Autodesk Inventor part; units mm, degrees
(part 2 of 3)
  arc A208 (-48.5424, -4.4941) -> (-48.5247, -4.6815) centre (0, 0) ccw
  arc A209 (-48.7692, -5.0892) -> (-48.5247, -4.6815) centre (-48.9228, -4.7199) ccw
  spline S104 degree 3 poles (-48.7692, -5.0892) (-49.5171, -5.4153) (-50.0527, -5.68) (-50.6439, -6.0168) knots 0 0 0 0 1 1 1 1
  line L312 (-48.7692, -5.0892) -> (-49.5171, -5.4153) construction
  line L313 (-49.5171, -5.4153) -> (-50.0527, -5.68) construction
  line L314 (-50.0527, -5.68) -> (-50.6439, -6.0168) construction
  arc A210 (-50.6439, -6.0168) -> (-50.5492, -6.7669) centre (0, 0) ccw
  spline S105 degree 3 poles (-50.5492, -6.7669) (-49.8928, -6.946) (-49.3082, -7.0693) (-48.5027, -7.1991) knots 0 0 0 0 1 1 1 1
  line L315 (-50.5492, -6.7669) -> (-49.8928, -6.946) construction
  line L316 (-49.8928, -6.946) -> (-49.3082, -7.0693) construction
  line L317 (-49.3082, -7.0693) -> (-48.5027, -7.1991) construction
  arc A211 (-48.1644, -7.5332) -> (-48.5027, -7.1991) centre (-48.5596, -7.595) ccw
  arc A212 (-48.1644, -7.5332) -> (-48.135, -7.7191) centre (0, 0) ccw
  arc A213 (-48.3535, -8.1414) -> (-48.135, -7.7191) centre (-48.5299, -7.7825) ccw
  spline S106 degree 3 poles (-48.3535, -8.1414) (-49.0794, -8.5138) (-49.5973, -8.8117) (-50.1662, -9.1848) knots 0 0 0 0 1 1 1 1
  line L318 (-48.3535, -8.1414) -> (-49.0794, -8.5138) construction
  line L319 (-49.0794, -8.5138) -> (-49.5973, -8.8117) construction
  line L320 (-49.5973, -8.8117) -> (-50.1662, -9.1848) construction
  arc A214 (-50.1662, -9.1848) -> (-50.0245, -9.9276) centre (0, 0) ccw
  spline S107 degree 3 poles (-50.0245, -9.9276) (-49.3582, -10.0651) (-48.767, -10.1514) (-47.955, -10.2304) knots 0 0 0 0 1 1 1 1
  line L321 (-50.0245, -9.9276) -> (-49.3582, -10.0651) construction
  line L322 (-49.3582, -10.0651) -> (-48.767, -10.1514) construction
  line L323 (-48.767, -10.1514) -> (-47.955, -10.2304) construction
  arc A215 (-47.5964, -10.5426) -> (-47.955, -10.2304) centre (-47.9869, -10.6291) ccw
  arc A216 (-47.5964, -10.5426) -> (-47.5553, -10.7263) centre (0, 0) ccw
  arc A217 (-47.7468, -11.1615) -> (-47.5553, -10.7263) centre (-47.9455, -10.8143) ccw
  spline S108 degree 3 poles (-47.7468, -11.1615) (-48.448, -11.5787) (-48.9462, -11.9085) (-49.4905, -12.3167) knots 0 0 0 0 1 1 1 1
  line L324 (-47.7468, -11.1615) -> (-48.448, -11.5787) construction
  line L325 (-48.448, -11.5787) -> (-48.9462, -11.9085) construction
  line L326 (-48.9462, -11.9085) -> (-49.4905, -12.3167) construction
  arc A218 (-49.4905, -12.3167) -> (-49.3024, -13.049) centre (0, 0) ccw
  spline S109 degree 3 poles (-49.3024, -13.049) (-48.6288, -13.1445) (-48.0334, -13.1935) (-47.218, -13.2213) knots 0 0 0 0 1 1 1 1
  line L327 (-49.3024, -13.049) -> (-48.6288, -13.1445) construction
  line L328 (-48.6288, -13.1445) -> (-48.0334, -13.1935) construction
  line L329 (-48.0334, -13.1935) -> (-47.218, -13.2213) construction
  arc A219 (-46.8405, -13.5104) -> (-47.218, -13.2213) centre (-47.2248, -13.6213) ccw
  arc A220 (-46.8405, -13.5104) -> (-46.788, -13.6912) centre (0, 0) ccw
  arc A221 (-46.9518, -14.1375) -> (-46.788, -13.6912) centre (-47.1719, -13.8035) ccw
  spline S110 degree 3 poles (-46.9518, -14.1375) (-47.6253, -14.5979) (-48.1018, -14.9584) (-48.6194, -15.3999) knots 0 0 0 0 1 1 1 1
  line L330 (-46.9518, -14.1375) -> (-47.6253, -14.5979) construction
  line L331 (-47.6253, -14.5979) -> (-48.1018, -14.9584) construction
  line L332 (-48.1018, -14.9584) -> (-48.6194, -15.3999) construction
  arc A222 (-48.6194, -15.3999) -> (-48.3858, -16.119) centre (0, 0) ccw
  spline S111 degree 3 poles (-48.3858, -16.119) (-47.7075, -16.172) (-47.1102, -16.1835) (-46.2946, -16.1601) knots 0 0 0 0 1 1 1 1
  line L333 (-48.3858, -16.119) -> (-47.7075, -16.172) construction
  line L334 (-47.7075, -16.172) -> (-47.1102, -16.1835) construction
  line L335 (-47.1102, -16.1835) -> (-46.2946, -16.1601) construction
  arc A223 (-45.8997, -16.4249) -> (-46.2946, -16.1601) centre (-46.2763, -16.5596) ccw
  arc A224 (-45.8997, -16.4249) -> (-45.836, -16.602) centre (0, 0) ccw
  arc A225 (-45.9714, -17.0578) -> (-45.836, -16.602) centre (-46.2121, -16.7382) ccw
  spline S112 degree 3 poles (-45.9714, -17.0578) (-46.6147, -17.5595) (-47.0677, -17.9492) (-47.5565, -18.4224) knots 0 0 0 0 1 1 1 1
  line L336 (-45.9714, -17.0578) -> (-46.6147, -17.5595) construction
  line L337 (-46.6147, -17.5595) -> (-47.0677, -17.9492) construction
  line L338 (-47.0677, -17.9492) -> (-47.5565, -18.4224) construction
  arc A226 (-47.5565, -18.4224) -> (-47.2782, -19.1254) centre (0, 0) ccw
  spline S113 degree 3 poles (-47.2782, -19.1254) (-46.5979, -19.1356) (-46.001, -19.1096) (-45.1886, -19.035) knots 0 0 0 0 1 1 1 1
  line L339 (-47.2782, -19.1254) -> (-46.5979, -19.1356) construction
  line L340 (-46.5979, -19.1356) -> (-46.001, -19.1096) construction
  line L341 (-46.001, -19.1096) -> (-45.1886, -19.035) construction
  arc A227 (-44.7778, -19.2745) -> (-45.1886, -19.035) centre (-45.1452, -19.4327) ccw
  arc A228 (-44.7778, -19.2745) -> (-44.7031, -19.4473) centre (0, 0) ccw
  arc A229 (-44.8097, -19.9107) -> (-44.7031, -19.4473) centre (-45.0699, -19.6069) ccw
  spline S114 degree 3 poles (-44.8097, -19.9107) (-45.4202, -20.4519) (-45.8478, -20.8692) (-46.3059, -21.3721) knots 0 0 0 0 1 1 1 1
  line L342 (-44.8097, -19.9107) -> (-45.4202, -20.4519) construction
  line L343 (-45.4202, -20.4519) -> (-45.8478, -20.8692) construction
  line L344 (-45.8478, -20.8692) -> (-46.3059, -21.3721) construction
  arc A230 (-46.3059, -21.3721) -> (-45.984, -22.0563) centre (0, 0) ccw
  spline S115 degree 3 poles (-45.984, -22.0563) (-45.3044, -22.0238) (-44.7103, -21.9604) (-43.9042, -21.8349) knots 0 0 0 0 1 1 1 1
  line L345 (-45.984, -22.0563) -> (-45.3044, -22.0238) construction
  line L346 (-45.3044, -22.0238) -> (-44.7103, -21.9604) construction
  line L347 (-44.7103, -21.9604) -> (-43.9042, -21.8349) construction
  arc A231 (-43.4792, -22.0481) -> (-43.9042, -21.8349) centre (-43.836, -22.229) ccw
  arc A232 (-43.4792, -22.0481) -> (-43.3938, -22.2159) centre (0, 0) ccw
  arc A233 (-43.471, -22.685) -> (-43.3938, -22.2159) centre (-43.7498, -22.3981) ccw
  spline S116 degree 3 poles (-43.471, -22.685) (-44.0464, -23.2635) (-44.4469, -23.7068) (-44.8726, -24.2375) knots 0 0 0 0 1 1 1 1
  line L348 (-43.471, -22.685) -> (-44.0464, -23.2635) construction
  line L349 (-44.0464, -23.2635) -> (-44.4469, -23.7068) construction
  line L350 (-44.4469, -23.7068) -> (-44.8726, -24.2375) construction
  arc A234 (-44.8726, -24.2375) -> (-44.5083, -24.9001) centre (0, 0) ccw
  spline S117 degree 3 poles (-44.5083, -24.9001) (-43.8322, -24.825) (-43.2432, -24.7244) (-42.4465, -24.5486) knots 0 0 0 0 1 1 1 1
  line L351 (-44.5083, -24.9001) -> (-43.8322, -24.825) construction
  line L352 (-43.8322, -24.825) -> (-43.2432, -24.7244) construction
  line L353 (-43.2432, -24.7244) -> (-42.4465, -24.5486) construction
  arc A235 (-42.009, -24.7347) -> (-42.4465, -24.5486) centre (-42.3537, -24.9377) ccw
  arc A236 (-42.009, -24.7347) -> (-41.9132, -24.8967) centre (0, 0) ccw
  arc A237 (-41.9609, -25.3698) -> (-41.9132, -24.8967) centre (-42.2571, -25.101) ccw
  spline S118 degree 3 poles (-41.9609, -25.3698) (-42.4987, -25.9832) (-42.8706, -26.4509) (-43.2622, -27.0072) knots 0 0 0 0 1 1 1 1
  line L354 (-41.9609, -25.3698) -> (-42.4987, -25.9832) construction
  line L355 (-42.4987, -25.9832) -> (-42.8706, -26.4509) construction
  line L356 (-42.8706, -26.4509) -> (-43.2622, -27.0072) construction
  arc A238 (-43.2622, -27.0072) -> (-42.857, -27.6457) centre (0, 0) ccw
  spline S119 degree 3 poles (-42.857, -27.6457) (-42.1869, -27.5283) (-41.6054, -27.3909) (-40.8213, -27.1654) knots 0 0 0 0 1 1 1 1
  line L357 (-42.857, -27.6457) -> (-42.1869, -27.5283) construction
  line L358 (-42.1869, -27.5283) -> (-41.6054, -27.3909) construction
  line L359 (-41.6054, -27.3909) -> (-40.8213, -27.1654) construction
  arc A239 (-40.373, -27.3237) -> (-40.8213, -27.1654) centre (-40.7043, -27.5479) ccw
  arc A240 (-40.373, -27.3237) -> (-40.2672, -27.4794) centre (0, 0) ccw
  arc A241 (-40.2851, -27.9545) -> (-40.2672, -27.4794) centre (-40.5976, -27.7048) ccw
  spline S120 degree 3 poles (-40.2851, -27.9545) (-40.7834, -28.6005) (-41.1252, -29.0905) (-41.481, -29.6704) knots 0 0 0 0 1 1 1 1
  line L360 (-40.2851, -27.9545) -> (-40.7834, -28.6005) construction
  line L361 (-40.7834, -28.6005) -> (-41.1252, -29.0905) construction
  line L362 (-41.1252, -29.0905) -> (-41.481, -29.6704) construction
  arc A242 (-41.481, -29.6704) -> (-41.0366, -30.2821) centre (0, 0) ccw
  spline S121 degree 3 poles (-41.0366, -30.2821) (-40.3751, -30.1229) (-39.8034, -29.9493) (-39.0351, -29.675) knots 0 0 0 0 1 1 1 1
  line L363 (-41.0366, -30.2821) -> (-40.3751, -30.1229) construction
  line L364 (-40.3751, -30.1229) -> (-39.8034, -29.9493) construction
  line L365 (-39.8034, -29.9493) -> (-39.0351, -29.675) construction
  arc A243 (-38.5777, -29.8048) -> (-39.0351, -29.675) centre (-38.8942, -30.0493) ccw
  arc A244 (-38.5777, -29.8048) -> (-38.4623, -29.9535) centre (0, 0) ccw
  arc A245 (-38.4503, -30.4288) -> (-38.4623, -29.9535) centre (-38.7779, -30.1993) ccw
  spline S122 degree 3 poles (-38.4503, -30.4288) (-38.9071, -31.1049) (-39.2174, -31.6154) (-39.5361, -32.2165) knots 0 0 0 0 1 1 1 1
  line L366 (-38.4503, -30.4288) -> (-38.9071, -31.1049) construction
  line L367 (-38.9071, -31.1049) -> (-39.2174, -31.6154) construction
  line L368 (-39.2174, -31.6154) -> (-39.5361, -32.2165) construction
  arc A246 (-39.5361, -32.2165) -> (-39.0542, -32.7991) centre (0, 0) ccw
  spline S123 degree 3 poles (-39.0542, -32.7991) (-38.404, -32.5986) (-37.8444, -32.3894) (-37.0947, -32.0674) knots 0 0 0 0 1 1 1 1
  line L369 (-39.0542, -32.7991) -> (-38.404, -32.5986) construction
  line L370 (-38.404, -32.5986) -> (-37.8444, -32.3894) construction
  line L371 (-37.8444, -32.3894) -> (-37.0947, -32.0674) construction
  arc A247 (-36.6301, -32.1683) -> (-37.0947, -32.0674) centre (-36.9306, -32.4322) ccw
  arc A248 (-36.6301, -32.1683) -> (-36.5056, -32.3095) centre (0, 0) ccw
  arc A249 (-36.4638, -32.7831) -> (-36.5056, -32.3095) centre (-36.8051, -32.5746) ccw
  spline S124 degree 3 poles (-36.4638, -32.7831) (-36.8772, -33.4865) (-37.1549, -34.0155) (-37.4352, -34.6354) knots 0 0 0 0 1 1 1 1
  line L372 (-36.4638, -32.7831) -> (-36.8772, -33.4865) construction
  line L373 (-36.8772, -33.4865) -> (-37.1549, -34.0155) construction
  line L374 (-37.1549, -34.0155) -> (-37.4352, -34.6354) construction
  arc A250 (-37.4352, -34.6354) -> (-36.9176, -35.1866) centre (0, 0) ccw
  spline S125 degree 3 poles (-36.9176, -35.1866) (-36.2814, -34.9457) (-35.7359, -34.7018) (-35.008, -34.3334) knots 0 0 0 0 1 1 1 1
  line L375 (-36.9176, -35.1866) -> (-36.2814, -34.9457) construction
  line L376 (-36.2814, -34.9457) -> (-35.7359, -34.7018) construction
  line L377 (-35.7359, -34.7018) -> (-35.008, -34.3334) construction
  arc A251 (-34.538, -34.4048) -> (-35.008, -34.3334) centre (-34.8213, -34.6871) ccw
  arc A252 (-34.538, -34.4048) -> (-34.4048, -34.538) centre (0, 0) ccw
  arc A253 (-34.3334, -35.008) -> (-34.4048, -34.538) centre (-34.6871, -34.8213) ccw
  spline S126 degree 3 poles (-34.3334, -35.008) (-34.7018, -35.7359) (-34.9457, -36.2814) (-35.1866, -36.9176) knots 0 0 0 0 1 1 1 1
  line L378 (-34.3334, -35.008) -> (-34.7018, -35.7359) construction
  line L379 (-34.7018, -35.7359) -> (-34.9457, -36.2814) construction
  line L380 (-34.9457, -36.2814) -> (-35.1866, -36.9176) construction
  arc A254 (-35.1866, -36.9176) -> (-34.6354, -37.4352) centre (0, 0) ccw
  spline S127 degree 3 poles (-34.6354, -37.4352) (-34.0155, -37.1549) (-33.4865, -36.8772) (-32.7831, -36.4638) knots 0 0 0 0 1 1 1 1
  line L381 (-34.6354, -37.4352) -> (-34.0155, -37.1549) construction
  line L382 (-34.0155, -37.1549) -> (-33.4865, -36.8772) construction
  line L383 (-33.4865, -36.8772) -> (-32.7831, -36.4638) construction
  arc A255 (-32.3095, -36.5056) -> (-32.7831, -36.4638) centre (-32.5746, -36.8051) ccw
  arc A256 (-32.3095, -36.5056) -> (-32.1683, -36.6301) centre (0, 0) ccw
  arc A257 (-32.0674, -37.0947) -> (-32.1683, -36.6301) centre (-32.4322, -36.9306) ccw
  spline S128 degree 3 poles (-32.0674, -37.0947) (-32.3894, -37.8444) (-32.5986, -38.404) (-32.7991, -39.0542) knots 0 0 0 0 1 1 1 1
  line L384 (-32.0674, -37.0947) -> (-32.3894, -37.8444) construction
  line L385 (-32.3894, -37.8444) -> (-32.5986, -38.404) construction
  line L386 (-32.5986, -38.404) -> (-32.7991, -39.0542) construction
  arc A258 (-32.7991, -39.0542) -> (-32.2165, -39.5361) centre (0, 0) ccw
  spline S129 degree 3 poles (-32.2165, -39.5361) (-31.6154, -39.2174) (-31.1049, -38.9071) (-30.4288, -38.4503) knots 0 0 0 0 1 1 1 1
  line L387 (-32.2165, -39.5361) -> (-31.6154, -39.2174) construction
  line L388 (-31.6154, -39.2174) -> (-31.1049, -38.9071) construction
  line L389 (-31.1049, -38.9071) -> (-30.4288, -38.4503) construction
  arc A259 (-29.9535, -38.4623) -> (-30.4288, -38.4503) centre (-30.1993, -38.7779) ccw
  arc A260 (-29.9535, -38.4623) -> (-29.8048, -38.5777) centre (0, 0) ccw
  arc A261 (-29.675, -39.0351) -> (-29.8048, -38.5777) centre (-30.0493, -38.8942) ccw
  spline S130 degree 3 poles (-29.675, -39.0351) (-29.9493, -39.8034) (-30.1229, -40.3751) (-30.2821, -41.0366) knots 0 0 0 0 1 1 1 1
  line L390 (-29.675, -39.0351) -> (-29.9493, -39.8034) construction
  line L391 (-29.9493, -39.8034) -> (-30.1229, -40.3751) construction
  line L392 (-30.1229, -40.3751) -> (-30.2821, -41.0366) construction
  arc A262 (-30.2821, -41.0366) -> (-29.6704, -41.481) centre (0, 0) ccw
  spline S131 degree 3 poles (-29.6704, -41.481) (-29.0905, -41.1252) (-28.6005, -40.7834) (-27.9545, -40.2851) knots 0 0 0 0 1 1 1 1
  line L393 (-29.6704, -41.481) -> (-29.0905, -41.1252) construction
  line L394 (-29.0905, -41.1252) -> (-28.6005, -40.7834) construction
  line L395 (-28.6005, -40.7834) -> (-27.9545, -40.2851) construction
  arc A263 (-27.4794, -40.2672) -> (-27.9545, -40.2851) centre (-27.7048, -40.5976) ccw
  arc A264 (-27.4794, -40.2672) -> (-27.3237, -40.373) centre (0, 0) ccw
  arc A265 (-27.1654, -40.8213) -> (-27.3237, -40.373) centre (-27.5479, -40.7043) ccw
  spline S132 degree 3 poles (-27.1654, -40.8213) (-27.3909, -41.6054) (-27.5283, -42.1869) (-27.6457, -42.857) knots 0 0 0 0 1 1 1 1
  line L396 (-27.1654, -40.8213) -> (-27.3909, -41.6054) construction
  line L397 (-27.3909, -41.6054) -> (-27.5283, -42.1869) construction
  line L398 (-27.5283, -42.1869) -> (-27.6457, -42.857) construction
  arc A266 (-27.6457, -42.857) -> (-27.0072, -43.2622) centre (0, 0) ccw
  spline S133 degree 3 poles (-27.0072, -43.2622) (-26.4509, -42.8706) (-25.9832, -42.4987) (-25.3698, -41.9609) knots 0 0 0 0 1 1 1 1
  line L399 (-27.0072, -43.2622) -> (-26.4509, -42.8706) construction
  line L400 (-26.4509, -42.8706) -> (-25.9832, -42.4987) construction
  line L401 (-25.9832, -42.4987) -> (-25.3698, -41.9609) construction
  arc A267 (-24.8967, -41.9132) -> (-25.3698, -41.9609) centre (-25.101, -42.2571) ccw
  arc A268 (-24.8967, -41.9132) -> (-24.7347, -42.009) centre (0, 0) ccw
  arc A269 (-24.5486, -42.4465) -> (-24.7347, -42.009) centre (-24.9377, -42.3537) ccw
  spline S134 degree 3 poles (-24.5486, -42.4465) (-24.7244, -43.2432) (-24.825, -43.8322) (-24.9001, -44.5083) knots 0 0 0 0 1 1 1 1
  line L402 (-24.5486, -42.4465) -> (-24.7244, -43.2432) construction
  line L403 (-24.7244, -43.2432) -> (-24.825, -43.8322) construction
  line L404 (-24.825, -43.8322) -> (-24.9001, -44.5083) construction
  arc A270 (-24.9001, -44.5083) -> (-24.2375, -44.8726) centre (0, 0) ccw
  spline S135 degree 3 poles (-24.2375, -44.8726) (-23.7068, -44.4469) (-23.2635, -44.0464) (-22.685, -43.471) knots 0 0 0 0 1 1 1 1
  line L405 (-24.2375, -44.8726) -> (-23.7068, -44.4469) construction
  line L406 (-23.7068, -44.4469) -> (-23.2635, -44.0464) construction
  line L407 (-23.2635, -44.0464) -> (-22.685, -43.471) construction
  arc A271 (-22.2159, -43.3938) -> (-22.685, -43.471) centre (-22.3981, -43.7498) ccw
  arc A272 (-22.2159, -43.3938) -> (-22.0481, -43.4792) centre (0, 0) ccw
  arc A273 (-21.8349, -43.9042) -> (-22.0481, -43.4792) centre (-22.229, -43.836) ccw
  spline S136 degree 3 poles (-21.8349, -43.9042) (-21.9604, -44.7103) (-22.0238, -45.3044) (-22.0563, -45.984) knots 0 0 0 0 1 1 1 1
  line L408 (-21.8349, -43.9042) -> (-21.9604, -44.7103) construction
  line L409 (-21.9604, -44.7103) -> (-22.0238, -45.3044) construction
  line L410 (-22.0238, -45.3044) -> (-22.0563, -45.984) construction
  arc A274 (-22.0563, -45.984) -> (-21.3721, -46.3059) centre (0, 0) ccw
  spline S137 degree 3 poles (-21.3721, -46.3059) (-20.8692, -45.8478) (-20.4519, -45.4202) (-19.9107, -44.8097) knots 0 0 0 0 1 1 1 1
  line L411 (-21.3721, -46.3059) -> (-20.8692, -45.8478) construction
  line L412 (-20.8692, -45.8478) -> (-20.4519, -45.4202) construction
  line L413 (-20.4519, -45.4202) -> (-19.9107, -44.8097) construction
  arc A275 (-19.4473, -44.7031) -> (-19.9107, -44.8097) centre (-19.6069, -45.0699) ccw
  arc A276 (-19.4473, -44.7031) -> (-19.2745, -44.7778) centre (0, 0) ccw
  arc A277 (-19.035, -45.1886) -> (-19.2745, -44.7778) centre (-19.4327, -45.1452) ccw
  spline S138 degree 3 poles (-19.035, -45.1886) (-19.1096, -46.001) (-19.1356, -46.5979) (-19.1254, -47.2782) knots 0 0 0 0 1 1 1 1
  line L414 (-19.035, -45.1886) -> (-19.1096, -46.001) construction
  line L415 (-19.1096, -46.001) -> (-19.1356, -46.5979) construction
  line L416 (-19.1356, -46.5979) -> (-19.1254, -47.2782) construction
  arc A278 (-19.1254, -47.2782) -> (-18.4224, -47.5565) centre (0, 0) ccw
  spline S139 degree 3 poles (-18.4224, -47.5565) (-17.9492, -47.0677) (-17.5595, -46.6147) (-17.0578, -45.9714) knots 0 0 0 0 1 1 1 1
  line L417 (-18.4224, -47.5565) -> (-17.9492, -47.0677) construction
  line L418 (-17.9492, -47.0677) -> (-17.5595, -46.6147) construction
  line L419 (-17.5595, -46.6147) -> (-17.0578, -45.9714) construction
  arc A279 (-16.602, -45.836) -> (-17.0578, -45.9714) centre (-16.7382, -46.2121) ccw
  arc A280 (-16.602, -45.836) -> (-16.4249, -45.8997) centre (0, 0) ccw
  arc A281 (-16.1601, -46.2946) -> (-16.4249, -45.8997) centre (-16.5596, -46.2763) ccw
  spline S140 degree 3 poles (-16.1601, -46.2946) (-16.1835, -47.1102) (-16.172, -47.7075) (-16.119, -48.3858) knots 0 0 0 0 1 1 1 1
  line L420 (-16.1601, -46.2946) -> (-16.1835, -47.1102) construction
  line L421 (-16.1835, -47.1102) -> (-16.172, -47.7075) construction
  line L422 (-16.172, -47.7075) -> (-16.119, -48.3858) construction
  arc A282 (-16.119, -48.3858) -> (-15.3999, -48.6194) centre (0, 0) ccw
  spline S141 degree 3 poles (-15.3999, -48.6194) (-14.9584, -48.1018) (-14.5979, -47.6253) (-14.1375, -46.9518) knots 0 0 0 0 1 1 1 1
  line L423 (-15.3999, -48.6194) -> (-14.9584, -48.1018) construction
  line L424 (-14.9584, -48.1018) -> (-14.5979, -47.6253) construction
  line L425 (-14.5979, -47.6253) -> (-14.1375, -46.9518) construction
  arc A283 (-13.6912, -46.788) -> (-14.1375, -46.9518) centre (-13.8035, -47.1719) ccw
  arc A284 (-13.6912, -46.788) -> (-13.5104, -46.8405) centre (0, 0) ccw
  arc A285 (-13.2213, -47.218) -> (-13.5104, -46.8405) centre (-13.6213, -47.2248) ccw
  spline S142 degree 3 poles (-13.2213, -47.218) (-13.1935, -48.0334) (-13.1445, -48.6288) (-13.049, -49.3024) knots 0 0 0 0 1 1 1 1
  line L426 (-13.2213, -47.218) -> (-13.1935, -48.0334) construction
  line L427 (-13.1935, -48.0334) -> (-13.1445, -48.6288) construction
  line L428 (-13.1445, -48.6288) -> (-13.049, -49.3024) construction
  arc A286 (-13.049, -49.3024) -> (-12.3167, -49.4905) centre (0, 0) ccw
  spline S143 degree 3 poles (-12.3167, -49.4905) (-11.9085, -48.9462) (-11.5787, -48.448) (-11.1615, -47.7468) knots 0 0 0 0 1 1 1 1
  line L429 (-12.3167, -49.4905) -> (-11.9085, -48.9462) construction
  line L430 (-11.9085, -48.9462) -> (-11.5787, -48.448) construction
  line L431 (-11.5787, -48.448) -> (-11.1615, -47.7468) construction
  arc A287 (-10.7263, -47.5553) -> (-11.1615, -47.7468) centre (-10.8143, -47.9455) ccw
  arc A288 (-10.7263, -47.5553) -> (-10.5426, -47.5964) centre (0, 0) ccw
  arc A289 (-10.2304, -47.955) -> (-10.5426, -47.5964) centre (-10.6291, -47.9869) ccw
  spline S144 degree 3 poles (-10.2304, -47.955) (-10.1514, -48.767) (-10.0651, -49.3582) (-9.9276, -50.0245) knots 0 0 0 0 1 1 1 1
  line L432 (-10.2304, -47.955) -> (-10.1514, -48.767) construction
  line L433 (-10.1514, -48.767) -> (-10.0651, -49.3582) construction
  line L434 (-10.0651, -49.3582) -> (-9.9276, -50.0245) construction
  arc A290 (-9.9276, -50.0245) -> (-9.1848, -50.1662) centre (0, 0) ccw
  spline S145 degree 3 poles (-9.1848, -50.1662) (-8.8117, -49.5973) (-8.5138, -49.0794) (-8.1414, -48.3535) knots 0 0 0 0 1 1 1 1
  line L435 (-9.1848, -50.1662) -> (-8.8117, -49.5973) construction
  line L436 (-8.8117, -49.5973) -> (-8.5138, -49.0794) construction
  line L437 (-8.5138, -49.0794) -> (-8.1414, -48.3535) construction
  arc A291 (-7.7191, -48.135) -> (-8.1414, -48.3535) centre (-7.7825, -48.5299) ccw
  arc A292 (-7.7191, -48.135) -> (-7.5332, -48.1644) centre (0, 0) ccw
  arc A293 (-7.1991, -48.5027) -> (-7.5332, -48.1644) centre (-7.595, -48.5596) ccw
  spline S146 degree 3 poles (-7.1991, -48.5027) (-7.0693, -49.3082) (-6.946, -49.8928) (-6.7669, -50.5492) knots 0 0 0 0 1 1 1 1
  line L438 (-7.1991, -48.5027) -> (-7.0693, -49.3082) construction
  line L439 (-7.0693, -49.3082) -> (-6.946, -49.8928) construction
  line L440 (-6.946, -49.8928) -> (-6.7669, -50.5492) construction
  arc A294 (-6.7669, -50.5492) -> (-6.0168, -50.6439) centre (0, 0) ccw
  spline S147 degree 3 poles (-6.0168, -50.6439) (-5.68, -50.0527) (-5.4153, -49.5171) (-5.0892, -48.7692) knots 0 0 0 0 1 1 1 1
  line L441 (-6.0168, -50.6439) -> (-5.68, -50.0527) construction
  line L442 (-5.68, -50.0527) -> (-5.4153, -49.5171) construction
  line L443 (-5.4153, -49.5171) -> (-5.0892, -48.7692) construction
  arc A295 (-4.6815, -48.5247) -> (-5.0892, -48.7692) centre (-4.7199, -48.9228) ccw
  arc A296 (-4.6815, -48.5247) -> (-4.4941, -48.5424) centre (0, 0) ccw
  arc A297 (-4.1394, -48.859) -> (-4.4941, -48.5424) centre (-4.5309, -48.9407) ccw
  spline S148 degree 3 poles (-4.1394, -48.859) (-3.9592, -49.6548) (-3.7995, -50.2305) (-3.5795, -50.8743) knots 0 0 0 0 1 1 1 1
  line L444 (-4.1394, -48.859) -> (-3.9592, -49.6548) construction
  line L445 (-3.9592, -49.6548) -> (-3.7995, -50.2305) construction
  line L446 (-3.7995, -50.2305) -> (-3.5795, -50.8743) construction
  arc A298 (-3.5795, -50.8743) -> (-2.8249, -50.9218) centre (0, 0) ccw
  spline S149 degree 3 poles (-2.8249, -50.9218) (-2.526, -50.3106) (-2.2954, -49.7595) (-2.0169, -48.9926) knots 0 0 0 0 1 1 1 1
  line L447 (-2.8249, -50.9218) -> (-2.526, -50.3106) construction
  line L448 (-2.526, -50.3106) -> (-2.2954, -49.7595) construction
  line L449 (-2.2954, -49.7595) -> (-2.0169, -48.9926) construction
  arc A299 (-1.6254, -48.7229) -> (-2.0169, -48.9926) centre (-1.6387, -49.1227) ccw
  arc A300 (-1.6254, -48.7229) -> (-1.4372, -48.7288) centre (0, 0) ccw
  arc A301 (-1.0633, -49.0225) -> (-1.4372, -48.7288) centre (-1.449, -49.1286) ccw
  spline S150 degree 3 poles (-1.0633, -49.0225) (-0.8336, -49.8054) (-0.638, -50.3699) (-0.3781, -50.9987) knots 0 0 0 0 1 1 1 1
  line L450 (-1.0633, -49.0225) -> (-0.8336, -49.8054) construction
  line L451 (-0.8336, -49.8054) -> (-0.638, -50.3699) construction
  line L452 (-0.638, -50.3699) -> (-0.3781, -50.9987) construction
  arc A302 (-0.3781, -50.9987) -> (0.3781, -50.9987) centre (0, 0) ccw
  spline S151 degree 3 poles (0.3781, -50.9987) (0.638, -50.3699) (0.8336, -49.8054) (1.0633, -49.0225) knots 0 0 0 0 1 1 1 1
  line L453 (0.3781, -50.9987) -> (0.638, -50.3699) construction
  line L454 (0.638, -50.3699) -> (0.8336, -49.8054) construction
  line L455 (0.8336, -49.8054) -> (1.0633, -49.0225) construction
  arc A303 (1.4372, -48.7288) -> (1.0633, -49.0225) centre (1.449, -49.1286) ccw
  arc A304 (1.4372, -48.7288) -> (1.6254, -48.7229) centre (0, 0) ccw
  arc A305 (2.0169, -48.9926) -> (1.6254, -48.7229) centre (1.6387, -49.1227) ccw
  spline S152 degree 3 poles (2.0169, -48.9926) (2.2954, -49.7595) (2.526, -50.3106) (2.8249, -50.9218) knots 0 0 0 0 1 1 1 1
  line L456 (2.0169, -48.9926) -> (2.2954, -49.7595) construction
  line L457 (2.2954, -49.7595) -> (2.526, -50.3106) construction
  line L458 (2.526, -50.3106) -> (2.8249, -50.9218) construction
  arc A306 (2.8249, -50.9218) -> (3.5795, -50.8743) centre (0, 0) ccw
  spline S153 degree 3 poles (3.5795, -50.8743) (3.7995, -50.2305) (3.9592, -49.6548) (4.1394, -48.859) knots 0 0 0 0 1 1 1 1
  line L459 (3.5795, -50.8743) -> (3.7995, -50.2305) construction
  line L460 (3.7995, -50.2305) -> (3.9592, -49.6548) construction
  line L461 (3.9592, -49.6548) -> (4.1394, -48.859) construction
  arc A307 (4.4941, -48.5424) -> (4.1394, -48.859) centre (4.5309, -48.9407) ccw
  arc A308 (4.4941, -48.5424) -> (4.6815, -48.5247) centre (0, 0) ccw
  arc A309 (5.0892, -48.7692) -> (4.6815, -48.5247) centre (4.7199, -48.9228) ccw
  spline S154 degree 3 poles (5.0892, -48.7692) (5.4153, -49.5171) (5.68, -50.0527) (6.0168, -50.6439) knots 0 0 0 0 1 1 1 1
  line L462 (5.0892, -48.7692) -> (5.4153, -49.5171) construction
  line L463 (5.4153, -49.5171) -> (5.68, -50.0527) construction
  line L464 (5.68, -50.0527) -> (6.0168, -50.6439) construction
  arc A310 (6.0168, -50.6439) -> (6.7669, -50.5492) centre (0, 0) ccw
  spline S155 degree 3 poles (6.7669, -50.5492) (6.946, -49.8928) (7.0693, -49.3082) (7.1991, -48.5027) knots 0 0 0 0 1 1 1 1
  line L465 (6.7669, -50.5492) -> (6.946, -49.8928) construction
  line L466 (6.946, -49.8928) -> (7.0693, -49.3082) construction
  line L467 (7.0693, -49.3082) -> (7.1991, -48.5027) construction
  arc A311 (7.5332, -48.1644) -> (7.1991, -48.5027) centre (7.595, -48.5596) ccw
  arc A312 (7.5332, -48.1644) -> (7.7191, -48.135) centre (0, 0) ccw
  arc A313 (8.1414, -48.3535) -> (7.7191, -48.135) centre (7.7825, -48.5299) ccw
  spline S156 degree 3 poles (8.1414, -48.3535) (8.5138, -49.0794) (8.8117, -49.5973) (9.1848, -50.1662) knots 0 0 0 0 1 1 1 1
  line L468 (8.1414, -48.3535) -> (8.5138, -49.0794) construction
  line L469 (8.5138, -49.0794) -> (8.8117, -49.5973) construction
  line L470 (8.8117, -49.5973) -> (9.1848, -50.1662) construction
  arc A314 (9.1848, -50.1662) -> (9.9276, -50.0245) centre (0, 0) ccw
  spline S157 degree 3 poles (9.9276, -50.0245) (10.0651, -49.3582) (10.1514, -48.767) (10.2304, -47.955) knots 0 0 0 0 1 1 1 1
  line L471 (9.9276, -50.0245) -> (10.0651, -49.3582) construction
  line L472 (10.0651, -49.3582) -> (10.1514, -48.767) construction
  line L473 (10.1514, -48.767) -> (10.2304, -47.955) construction
  arc A315 (10.5426, -47.5964) -> (10.2304, -47.955) centre (10.6291, -47.9869) ccw
  arc A316 (10.5426, -47.5964) -> (10.7263, -47.5553) centre (0, 0) ccw
  arc A317 (11.1615, -47.7468) -> (10.7263, -47.5553) centre (10.8143, -47.9455) ccw
  spline S158 degree 3 poles (11.1615, -47.7468) (11.5787, -48.448) (11.9085, -48.9462) (12.3167, -49.4905) knots 0 0 0 0 1 1 1 1
  line L474 (11.1615, -47.7468) -> (11.5787, -48.448) construction
  line L475 (11.5787, -48.448) -> (11.9085, -48.9462) construction
  line L476 (11.9085, -48.9462) -> (12.3167, -49.4905) construction
  arc A318 (12.3167, -49.4905) -> (13.049, -49.3024) centre (0, 0) ccw
  spline S159 degree 3 poles (13.049, -49.3024) (13.1445, -48.6288) (13.1935, -48.0334) (13.2213, -47.218) knots 0 0 0 0 1 1 1 1
  line L477 (13.049, -49.3024) -> (13.1445, -48.6288) construction
  line L478 (13.1445, -48.6288) -> (13.1935, -48.0334) construction
  line L479 (13.1935, -48.0334) -> (13.2213, -47.218) construction
  arc A319 (13.5104, -46.8405) -> (13.2213, -47.218) centre (13.6213, -47.2248) ccw
  arc A320 (13.5104, -46.8405) -> (13.6912, -46.788) centre (0, 0) ccw
  arc A321 (14.1375, -46.9518) -> (13.6912, -46.788) centre (13.8035, -47.1719) ccw
  spline S160 degree 3 poles (14.1375, -46.9518) (14.5979, -47.6253) (14.9584, -48.1018) (15.3999, -48.6194) knots 0 0 0 0 1 1 1 1
  line L480 (14.1375, -46.9518) -> (14.5979, -47.6253) construction
  line L481 (14.5979, -47.6253) -> (14.9584, -48.1018) construction
  line L482 (14.9584, -48.1018) -> (15.3999, -48.6194) construction
  arc A322 (15.3999, -48.6194) -> (16.119, -48.3858) centre (0, 0) ccw
  spline S161 degree 3 poles (16.119, -48.3858) (16.172, -47.7075) (16.1835, -47.1102) (16.1601, -46.2946) knots 0 0 0 0 1 1 1 1
  line L483 (16.119, -48.3858) -> (16.172, -47.7075) construction
  line L484 (16.172, -47.7075) -> (16.1835, -47.1102) construction
  line L485 (16.1835, -47.1102) -> (16.1601, -46.2946) construction
  arc A323 (16.4249, -45.8997) -> (16.1601, -46.2946) centre (16.5596, -46.2763) ccw
  arc A324 (16.4249, -45.8997) -> (16.602, -45.836) centre (0, 0) ccw
  arc A325 (17.0578, -45.9714) -> (16.602, -45.836) centre (16.7382, -46.2121) ccw
  spline S162 degree 3 poles (17.0578, -45.9714) (17.5595, -46.6147) (17.9492, -47.0677) (18.4224, -47.5565) knots 0 0 0 0 1 1 1 1
  line L486 (17.0578, -45.9714) -> (17.5595, -46.6147) construction
  line L487 (17.5595, -46.6147) -> (17.9492, -47.0677) construction
  line L488 (17.9492, -47.0677) -> (18.4224, -47.5565) construction
  arc A326 (18.4224, -47.5565) -> (19.1254, -47.2782) centre (0, 0) ccw
  spline S163 degree 3 poles (19.1254, -47.2782) (19.1356, -46.5979) (19.1096, -46.001) (19.035, -45.1886) knots 0 0 0 0 1 1 1 1
  line L489 (19.1254, -47.2782) -> (19.1356, -46.5979) construction
  line L490 (19.1356, -46.5979) -> (19.1096, -46.001) construction
  line L491 (19.1096, -46.001) -> (19.035, -45.1886) construction
  arc A327 (19.2745, -44.7778) -> (19.035, -45.1886) centre (19.4327, -45.1452) ccw
  arc A328 (19.2745, -44.7778) -> (19.4473, -44.7031) centre (0, 0) ccw
  arc A329 (19.9107, -44.8097) -> (19.4473, -44.7031) centre (19.6069, -45.0699) ccw
  spline S164 degree 3 poles (19.9107, -44.8097) (20.4519, -45.4202) (20.8692, -45.8478) (21.3721, -46.3059) knots 0 0 0 0 1 1 1 1
  line L492 (19.9107, -44.8097) -> (20.4519, -45.4202) construction
  line L493 (20.4519, -45.4202) -> (20.8692, -45.8478) construction
  line L494 (20.8692, -45.8478) -> (21.3721, -46.3059) construction
  arc A330 (21.3721, -46.3059) -> (22.0563, -45.984) centre (0, 0) ccw
  spline S165 degree 3 poles (22.0563, -45.984) (22.0238, -45.3044) (21.9604, -44.7103) (21.8349, -43.9042) knots 0 0 0 0 1 1 1 1
  line L495 (22.0563, -45.984) -> (22.0238, -45.3044) construction
  line L496 (22.0238, -45.3044) -> (21.9604, -44.7103) construction
  line L497 (21.9604, -44.7103) -> (21.8349, -43.9042) construction
  arc A331 (22.0481, -43.4792) -> (21.8349, -43.9042) centre (22.229, -43.836) ccw
  arc A332 (22.0481, -43.4792) -> (22.2159, -43.3938) centre (0, 0) ccw
  arc A333 (22.685, -43.471) -> (22.2159, -43.3938) centre (22.3981, -43.7498) ccw
  spline S166 degree 3 poles (22.685, -43.471) (23.2635, -44.0464) (23.7068, -44.4469) (24.2375, -44.8726) knots 0 0 0 0 1 1 1 1
  line L498 (22.685, -43.471) -> (23.2635, -44.0464) construction
  line L499 (23.2635, -44.0464) -> (23.7068, -44.4469) construction
  line L500 (23.7068, -44.4469) -> (24.2375, -44.8726) construction
  arc A334 (24.2375, -44.8726) -> (24.9001, -44.5083) centre (0, 0) ccw
  spline S167 degree 3 poles (24.9001, -44.5083) (24.825, -43.8322) (24.7244, -43.2432) (24.5486, -42.4465) knots 0 0 0 0 1 1 1 1
  line L501 (24.9001, -44.5083) -> (24.825, -43.8322) construction
  line L502 (24.825, -43.8322) -> (24.7244, -43.2432) construction
  line L503 (24.7244, -43.2432) -> (24.5486, -42.4465) construction
  arc A335 (24.7347, -42.009) -> (24.5486, -42.4465) centre (24.9377, -42.3537) ccw
  arc A336 (24.7347, -42.009) -> (24.8967, -41.9132) centre (0, 0) ccw
  arc A337 (25.3698, -41.9609) -> (24.8967, -41.9132) centre (25.101, -42.2571) ccw
  spline S168 degree 3 poles (25.3698, -41.9609) (25.9832, -42.4987) (26.4509, -42.8706) (27.0072, -43.2622) knots 0 0 0 0 1 1 1 1
  line L504 (25.3698, -41.9609) -> (25.9832, -42.4987) construction
  line L505 (25.9832, -42.4987) -> (26.4509, -42.8706) construction
  line L506 (26.4509, -42.8706) -> (27.0072, -43.2622) construction
  arc A338 (27.0072, -43.2622) -> (27.6457, -42.857) centre (0, 0) ccw
  spline S169 degree 3 poles (27.6457, -42.857) (27.5283, -42.1869) (27.3909, -41.6054) (27.1654, -40.8213) knots 0 0 0 0 1 1 1 1
  line L507 (27.6457, -42.857) -> (27.5283, -42.1869) construction
  line L508 (27.5283, -42.1869) -> (27.3909, -41.6054) construction
  line L509 (27.3909, -41.6054) -> (27.1654, -40.8213) construction
  arc A339 (27.3237, -40.373) -> (27.1654, -40.8213) centre (27.5479, -40.7043) ccw
  arc A340 (27.3237, -40.373) -> (27.4794, -40.2672) centre (0, 0) ccw
  arc A341 (27.9545, -40.2851) -> (27.4794, -40.2672) centre (27.7048, -40.5976) ccw
  spline S170 degree 3 poles (27.9545, -40.2851) (28.6005, -40.7834) (29.0905, -41.1252) (29.6704, -41.481) knots 0 0 0 0 1 1 1 1
  line L510 (27.9545, -40.2851) -> (28.6005, -40.7834) construction
  line L511 (28.6005, -40.7834) -> (29.0905, -41.1252) construction
  line L512 (29.0905, -41.1252) -> (29.6704, -41.481) construction
  arc A342 (29.6704, -41.481) -> (30.2821, -41.0366) centre (0, 0) ccw
  spline S171 degree 3 poles (30.2821, -41.0366) (30.1229, -40.3751) (29.9493, -39.8034) (29.675, -39.0351) knots 0 0 0 0 1 1 1 1
  line L513 (30.2821, -41.0366) -> (30.1229, -40.3751) construction
  line L514 (30.1229, -40.3751) -> (29.9493, -39.8034) construction
  line L515 (29.9493, -39.8034) -> (29.675, -39.0351) construction
  arc A343 (29.8048, -38.5777) -> (29.675, -39.0351) centre (30.0493, -38.8942) ccw
  arc A344 (29.8048, -38.5777) -> (29.9535, -38.4623) centre (0, 0) ccw
  arc A345 (30.4288, -38.4503) -> (29.9535, -38.4623) centre (30.1993, -38.7779) ccw
  spline S172 degree 3 poles (30.4288, -38.4503) (31.1049, -38.9071) (31.6154, -39.2174) (32.2165, -39.5361) knots 0 0 0 0 1 1 1 1
  line L516 (30.4288, -38.4503) -> (31.1049, -38.9071) construction
  line L517 (31.1049, -38.9071) -> (31.6154, -39.2174) construction
  line L518 (31.6154, -39.2174) -> (32.2165, -39.5361) construction
  arc A346 (32.2165, -39.5361) -> (32.7991, -39.0542) centre (0, 0) ccw
  spline S173 degree 3 poles (32.7991, -39.0542) (32.5986, -38.404) (32.3894, -37.8444) (32.0674, -37.0947) knots 0 0 0 0 1 1 1 1
  line L519 (32.7991, -39.0542) -> (32.5986, -38.404) construction
  line L520 (32.5986, -38.404) -> (32.3894, -37.8444) construction
  line L521 (32.3894, -37.8444) -> (32.0674, -37.0947) construction
  arc A347 (32.1683, -36.6301) -> (32.0674, -37.0947) centre (32.4322, -36.9306) ccw
  arc A348 (32.1683, -36.6301) -> (32.3095, -36.5056) centre (0, 0) ccw
  arc A349 (32.7831, -36.4638) -> (32.3095, -36.5056) centre (32.5746, -36.8051) ccw
  spline S174 degree 3 poles (32.7831, -36.4638) (33.4865, -36.8772) (34.0155, -37.1549) (34.6354, -37.4352) knots 0 0 0 0 1 1 1 1
  line L522 (32.7831, -36.4638) -> (33.4865, -36.8772) construction
  line L523 (33.4865, -36.8772) -> (34.0155, -37.1549) construction
  line L524 (34.0155, -37.1549) -> (34.6354, -37.4352) construction
  arc A350 (34.6354, -37.4352) -> (35.1866, -36.9176) centre (0, 0) ccw
  spline S175 degree 3 poles (35.1866, -36.9176) (34.9457, -36.2814) (34.7018, -35.7359) (34.3334, -35.008) knots 0 0 0 0 1 1 1 1
  line L525 (35.1866, -36.9176) -> (34.9457, -36.2814) construction
  line L526 (34.9457, -36.2814) -> (34.7018, -35.7359) construction
  line L527 (34.7018, -35.7359) -> (34.3334, -35.008) construction
  arc A351 (34.4048, -34.538) -> (34.3334, -35.008) centre (34.6871, -34.8213) ccw
  arc A352 (34.4048, -34.538) -> (34.538, -34.4048) centre (0, 0) ccw
  arc A353 (35.008, -34.3334) -> (34.538, -34.4048) centre (34.8213, -34.6871) ccw
  spline S176 degree 3 poles (35.008, -34.3334) (35.7359, -34.7018) (36.2814, -34.9457) (36.9176, -35.1866) knots 0 0 0 0 1 1 1 1
  line L528 (35.008, -34.3334) -> (35.7359, -34.7018) construction
  line L529 (35.7359, -34.7018) -> (36.2814, -34.9457) construction
  line L530 (36.2814, -34.9457) -> (36.9176, -35.1866) construction
  arc A354 (36.9176, -35.1866) -> (37.4352, -34.6354) centre (0, 0) ccw
  spline S177 degree 3 poles (37.4352, -34.6354) (37.1549, -34.0155) (36.8772, -33.4865) (36.4638, -32.7831) knots 0 0 0 0 1 1 1 1
  line L531 (37.4352, -34.6354) -> (37.1549, -34.0155) construction
  line L532 (37.1549, -34.0155) -> (36.8772, -33.4865) construction
  line L533 (36.8772, -33.4865) -> (36.4638, -32.7831) construction
  arc A355 (36.5056, -32.3095) -> (36.4638, -32.7831) centre (36.8051, -32.5746) ccw
  arc A356 (36.5056, -32.3095) -> (36.6301, -32.1683) centre (0, 0) ccw
  arc A357 (37.0947, -32.0674) -> (36.6301, -32.1683) centre (36.9306, -32.4322) ccw
  spline S178 degree 3 poles (37.0947, -32.0674) (37.8444, -32.3894) (38.404, -32.5986) (39.0542, -32.7991) knots 0 0 0 0 1 1 1 1
  line L534 (37.0947, -32.0674) -> (37.8444, -32.3894) construction
  line L535 (37.8444, -32.3894) -> (38.404, -32.5986) construction
  line L536 (38.404, -32.5986) -> (39.0542, -32.7991) construction
  arc A358 (39.0542, -32.7991) -> (39.5361, -32.2165) centre (0, 0) ccw
  spline S179 degree 3 poles (39.5361, -32.2165) (39.2174, -31.6154) (38.9071, -31.1049) (38.4503, -30.4288) knots 0 0 0 0 1 1 1 1
  line L537 (39.5361, -32.2165) -> (39.2174, -31.6154) construction
  line L538 (39.2174, -31.6154) -> (38.9071, -31.1049) construction
  line L539 (38.9071, -31.1049) -> (38.4503, -30.4288) construction
  arc A359 (38.4623, -29.9535) -> (38.4503, -30.4288) centre (38.7779, -30.1993) ccw
  arc A360 (38.4623, -29.9535) -> (38.5777, -29.8048) centre (0, 0) ccw
  arc A361 (39.0351, -29.675) -> (38.5777, -29.8048) centre (38.8942, -30.0493) ccw
  spline S180 degree 3 poles (39.0351, -29.675) (39.8034, -29.9493) (40.3751, -30.1229) (41.0366, -30.2821) knots 0 0 0 0 1 1 1 1
  line L540 (39.0351, -29.675) -> (39.8034, -29.9493) construction
  line L541 (39.8034, -29.9493) -> (40.3751, -30.1229) construction
  line L542 (40.3751, -30.1229) -> (41.0366, -30.2821) construction
  arc A362 (41.0366, -30.2821) -> (41.481, -29.6704) centre (0, 0) ccw
  spline S181 degree 3 poles (41.481, -29.6704) (41.1252, -29.0905) (40.7834, -28.6005) (40.2851, -27.9545) knots 0 0 0 0 1 1 1 1
  line L543 (41.481, -29.6704) -> (41.1252, -29.0905) construction
  line L544 (41.1252, -29.0905) -> (40.7834, -28.6005) construction
  line L545 (40.7834, -28.6005) -> (40.2851, -27.9545) construction
  arc A363 (40.2672, -27.4794) -> (40.2851, -27.9545) centre (40.5976, -27.7048) ccw
  arc A364 (40.2672, -27.4794) -> (40.373, -27.3237) centre (0, 0) ccw
  arc A365 (40.8213, -27.1654) -> (40.373, -27.3237) centre (40.7043, -27.5479) ccw
  spline S182 degree 3 poles (40.8213, -27.1654) (41.6054, -27.3909) (42.1869, -27.5283) (42.857, -27.6457) knots 0 0 0 0 1 1 1 1
  line L546 (40.8213, -27.1654) -> (41.6054, -27.3909) construction
  line L547 (41.6054, -27.3909) -> (42.1869, -27.5283) construction
  line L548 (42.1869, -27.5283) -> (42.857, -27.6457) construction
  arc A366 (42.857, -27.6457) -> (43.2622, -27.0072) centre (0, 0) ccw
  spline S183 degree 3 poles (43.2622, -27.0072) (42.8706, -26.4509) (42.4987, -25.9832) (41.9609, -25.3698) knots 0 0 0 0 1 1 1 1
  line L549 (43.2622, -27.0072) -> (42.8706, -26.4509) construction
  line L550 (42.8706, -26.4509) -> (42.4987, -25.9832) construction
  line L551 (42.4987, -25.9832) -> (41.9609, -25.3698) construction
  arc A367 (41.9132, -24.8967) -> (41.9609, -25.3698) centre (42.2571, -25.101) ccw
  arc A368 (41.9132, -24.8967) -> (42.009, -24.7347) centre (0, 0) ccw
  arc A369 (42.4465, -24.5486) -> (42.009, -24.7347) centre (42.3537, -24.9377) ccw
  spline S184 degree 3 poles (42.4465, -24.5486) (43.2432, -24.7244) (43.8322, -24.825) (44.5083, -24.9001) knots 0 0 0 0 1 1 1 1
  line L552 (42.4465, -24.5486) -> (43.2432, -24.7244) construction
  line L553 (43.2432, -24.7244) -> (43.8322, -24.825) construction
  line L554 (43.8322, -24.825) -> (44.5083, -24.9001) construction
  arc A370 (44.5083, -24.9001) -> (44.8726, -24.2375) centre (0, 0) ccw
  spline S185 degree 3 poles (44.8726, -24.2375) (44.4469, -23.7068) (44.0464, -23.2635) (43.471, -22.685) knots 0 0 0 0 1 1 1 1
  line L555 (44.8726, -24.2375) -> (44.4469, -23.7068) construction
  line L556 (44.4469, -23.7068) -> (44.0464, -23.2635) construction
  line L557 (44.0464, -23.2635) -> (43.471, -22.685) construction
  arc A371 (43.3938, -22.2159) -> (43.471, -22.685) centre (43.7498, -22.3981) ccw
  arc A372 (43.3938, -22.2159) -> (43.4792, -22.0481) centre (0, 0) ccw
  arc A373 (43.9042, -21.8349) -> (43.4792, -22.0481) centre (43.836, -22.229) ccw
  spline S186 degree 3 poles (43.9042, -21.8349) (44.7103, -21.9604) (45.3044, -22.0238) (45.984, -22.0563) knots 0 0 0 0 1 1 1 1
  line L558 (43.9042, -21.8349) -> (44.7103, -21.9604) construction
  line L559 (44.7103, -21.9604) -> (45.3044, -22.0238) construction
  line L560 (45.3044, -22.0238) -> (45.984, -22.0563) construction
  arc A374 (45.984, -22.0563) -> (46.3059, -21.3721) centre (0, 0) ccw
  spline S187 degree 3 poles (46.3059, -21.3721) (45.8478, -20.8692) (45.4202, -20.4519) (44.8097, -19.9107) knots 0 0 0 0 1 1 1 1
  line L561 (46.3059, -21.3721) -> (45.8478, -20.8692) construction
  line L562 (45.8478, -20.8692) -> (45.4202, -20.4519) construction
  line L563 (45.4202, -20.4519) -> (44.8097, -19.9107) construction
  arc A375 (44.7031, -19.4473) -> (44.8097, -19.9107) centre (45.0699, -19.6069) ccw
  arc A376 (44.7031, -19.4473) -> (44.7778, -19.2745) centre (0, 0) ccw
  arc A377 (45.1886, -19.035) -> (44.7778, -19.2745) centre (45.1452, -19.4327) ccw
  spline S188 degree 3 poles (45.1886, -19.035) (46.001, -19.1096) (46.5979, -19.1356) (47.2782, -19.1254) knots 0 0 0 0 1 1 1 1
  line L564 (45.1886, -19.035) -> (46.001, -19.1096) construction
  line L565 (46.001, -19.1096) -> (46.5979, -19.1356) construction
  line L566 (46.5979, -19.1356) -> (47.2782, -19.1254) construction
  arc A378 (47.2782, -19.1254) -> (47.5565, -18.4224) centre (0, 0) ccw
  spline S189 degree 3 poles (47.5565, -18.4224) (47.0677, -17.9492) (46.6147, -17.5595) (45.9714, -17.0578) knots 0 0 0 0 1 1 1 1
  line L567 (47.5565, -18.4224) -> (47.0677, -17.9492) construction
  line L568 (47.0677, -17.9492) -> (46.6147, -17.5595) construction
  line L569 (46.6147, -17.5595) -> (45.9714, -17.0578) construction
  arc A379 (45.836, -16.602) -> (45.9714, -17.0578) centre (46.2121, -16.7382) ccw
  arc A380 (45.836, -16.602) -> (45.8997, -16.4249) centre (0, 0) ccw
  arc A381 (46.2946, -16.1601) -> (45.8997, -16.4249) centre (46.2763, -16.5596) ccw
  spline S190 degree 3 poles (46.2946, -16.1601) (47.1102, -16.1835) (47.7075, -16.172) (48.3858, -16.119) knots 0 0 0 0 1 1 1 1
  line L570 (46.2946, -16.1601) -> (47.1102, -16.1835) construction
  line L571 (47.1102, -16.1835) -> (47.7075, -16.172) construction
  line L572 (47.7075, -16.172) -> (48.3858, -16.119) construction
  arc A382 (48.3858, -16.119) -> (48.6194, -15.3999) centre (0, 0) ccw
  spline S191 degree 3 poles (48.6194, -15.3999) (48.1018, -14.9584) (47.6253, -14.5979) (46.9518, -14.1375) knots 0 0 0 0 1 1 1 1
  line L573 (48.6194, -15.3999) -> (48.1018, -14.9584) construction
  line L574 (48.1018, -14.9584) -> (47.6253, -14.5979) construction
  line L575 (47.6253, -14.5979) -> (46.9518, -14.1375) construction
  arc A383 (46.788, -13.6912) -> (46.9518, -14.1375) centre (47.1719, -13.8035) ccw
  arc A384 (46.788, -13.6912) -> (46.8405, -13.5104) centre (0, 0) ccw
  arc A385 (47.218, -13.2213) -> (46.8405, -13.5104) centre (47.2248, -13.6213) ccw
  spline S192 degree 3 poles (47.218, -13.2213) (48.0334, -13.1935) (48.6288, -13.1445) (49.3024, -13.049) knots 0 0 0 0 1 1 1 1
  line L576 (47.218, -13.2213) -> (48.0334, -13.1935) construction
  line L577 (48.0334, -13.1935) -> (48.6288, -13.1445) construction
  line L578 (48.6288, -13.1445) -> (49.3024, -13.049) construction
  arc A386 (49.3024, -13.049) -> (49.4905, -12.3167) centre (0, 0) ccw
  spline S193 degree 3 poles (49.4905, -12.3167) (48.9462, -11.9085) (48.448, -11.5787) (47.7468, -11.1615) knots 0 0 0 0 1 1 1 1
  line L579 (49.4905, -12.3167) -> (48.9462, -11.9085) construction
  line L580 (48.9462, -11.9085) -> (48.448, -11.5787) construction
  line L581 (48.448, -11.5787) -> (47.7468, -11.1615) construction
  arc A387 (47.5553, -10.7263) -> (47.7468, -11.1615) centre (47.9455, -10.8143) ccw
  arc A388 (47.5553, -10.7263) -> (47.5964, -10.5426) centre (0, 0) ccw
  arc A389 (47.955, -10.2304) -> (47.5964, -10.5426) centre (47.9869, -10.6291) ccw
  spline S194 degree 3 poles (47.955, -10.2304) (48.767, -10.1514) (49.3582, -10.0651) (50.0245, -9.9276) knots 0 0 0 0 1 1 1 1
  line L582 (47.955, -10.2304) -> (48.767, -10.1514) construction
  line L583 (48.767, -10.1514) -> (49.3582, -10.0651) construction
  line L584 (49.3582, -10.0651) -> (50.0245, -9.9276) construction
  arc A390 (50.0245, -9.9276) -> (50.1662, -9.1848) centre (0, 0) ccw
  spline S195 degree 3 poles (50.1662, -9.1848) (49.5973, -8.8117) (49.0794, -8.5138) (48.3535, -8.1414) knots 0 0 0 0 1 1 1 1
  line L585 (50.1662, -9.1848) -> (49.5973, -8.8117) construction
  line L586 (49.5973, -8.8117) -> (49.0794, -8.5138) construction
  line L587 (49.0794, -8.5138) -> (48.3535, -8.1414) construction
  arc A391 (48.135, -7.7191) -> (48.3535, -8.1414) centre (48.5299, -7.7825) ccw
  arc A392 (48.135, -7.7191) -> (48.1644, -7.5332) centre (0, 0) ccw
  arc A393 (48.5027, -7.1991) -> (48.1644, -7.5332) centre (48.5596, -7.595) ccw
  spline S196 degree 3 poles (48.5027, -7.1991) (49.3082, -7.0693) (49.8928, -6.946) (50.5492, -6.7669) knots 0 0 0 0 1 1 1 1
  line L588 (48.5027, -7.1991) -> (49.3082, -7.0693) construction
  line L589 (49.3082, -7.0693) -> (49.8928, -6.946) construction
  line L590 (49.8928, -6.946) -> (50.5492, -6.7669) construction
  arc A394 (50.5492, -6.7669) -> (50.6439, -6.0168) centre (0, 0) ccw
  spline S197 degree 3 poles (50.6439, -6.0168) (50.0527, -5.68) (49.5171, -5.4153) (48.7692, -5.0892) knots 0 0 0 0 1 1 1 1
  line L591 (50.6439, -6.0168) -> (50.0527, -5.68) construction
  line L592 (50.0527, -5.68) -> (49.5171, -5.4153) construction
  line L593 (49.5171, -5.4153) -> (48.7692, -5.0892) construction
  arc A395 (48.5247, -4.6815) -> (48.7692, -5.0892) centre (48.9228, -4.7199) ccw
  arc A396 (48.5247, -4.6815) -> (48.5424, -4.4941) centre (0, 0) ccw
  arc A397 (48.859, -4.1394) -> (48.5424, -4.4941) centre (48.9407, -4.5309) ccw
  spline S198 degree 3 poles (48.859, -4.1394) (49.6548, -3.9592) (50.2305, -3.7995) (50.8743, -3.5795) knots 0 0 0 0 1 1 1 1
  line L594 (48.859, -4.1394) -> (49.6548, -3.9592) construction
  line L595 (49.6548, -3.9592) -> (50.2305, -3.7995) construction
  line L596 (50.2305, -3.7995) -> (50.8743, -3.5795) construction
  arc A398 (50.8743, -3.5795) -> (50.9218, -2.8249) centre (0, 0) ccw
  spline S199 degree 3 poles (50.9218, -2.8249) (50.3106, -2.526) (49.7595, -2.2954) (48.9926, -2.0169) knots 0 0 0 0 1 1 1 1
  line L597 (50.9218, -2.8249) -> (50.3106, -2.526) construction
  line L598 (50.3106, -2.526) -> (49.7595, -2.2954) construction
  line L599 (49.7595, -2.2954) -> (48.9926, -2.0169) construction
  arc A399 (48.7229, -1.6254) -> (48.9926, -2.0169) centre (49.1227, -1.6387) ccw
  point P0 (48.8646, -4.1381)
  point P1 (48.9926, -2.0169)
  point P2 (48.7229, -1.6254)
  point P3 (48.7288, -1.4372)
  point P4 (49.028, -1.0617)
  point P5 (49.0225, 1.0633)
  point P6 (48.7288, 1.4372)
  point P7 (48.7229, 1.6254)
  point P8 (48.9979, 2.0189)
  point P9 (48.859, 4.1394)
  point P10 (48.5424, 4.4941)
  point P11 (48.5247, 4.6815)
  point P12 (48.7692, 5.0892)
  point P13 (50.6439, 6.0168)
  point P14 (48.1644, 7.5332)
  point P15 (48.135, 7.7191)
  point P16 (48.3585, 8.144)
  point P17 (50.1662, 9.1848)
  point P18 (47.5964, 10.5426)
  point P19 (47.5553, 10.7263)
  point P20 (47.7517, 11.1644)
  point P21 (46.8405, 13.5104)
  point P22 (46.788, 13.6912)
  point P23 (46.9565, 14.1407)
  point P24 (46.2946, 16.1601)
  point P25 (45.8997, 16.4249)
  point P26 (45.836, 16.602)
  point P27 (45.9759, 17.0612)
  point P28 (44.7778, 19.2745)
  point P29 (44.7031, 19.4473)
  point P30 (44.8139, 19.9144)
  point P31 (46.3059, 21.3721)
  point P32 (43.9042, 21.8349)
  point P33 (43.4792, 22.0481)
  point P34 (43.3938, 22.2159)
  point P35 (44.8726, 24.2375)
  point P36 (42.009, 24.7347)
  point P37 (41.9132, 24.8967)
  point P38 (41.9646, 25.3741)
  point P39 (43.2622, 27.0072)
  point P40 (40.8213, 27.1654)
  point P41 (40.373, 27.3237)
  point P42 (40.2672, 27.4794)
  point P43 (40.2885, 27.959)
  point P44 (41.481, 29.6704)
  point P45 (38.5777, 29.8048)
  point P46 (38.4623, 29.9535)
  point P47 (38.4535, 30.4336)
  point P48 (39.5361, 32.2165)
  point P49 (37.0947, 32.0674)
  point P50 (36.6301, 32.1683)
  point P51 (36.5056, 32.3095)
  point P52 (36.4667, 32.788)
  point P53 (37.4352, 34.6354)
  point P54 (34.5379, 34.4048)
  point P55 (34.4048, 34.5379)
  point P56 (34.3359, 35.0131)
  point P57 (32.3095, 36.5056)
  point P58 (32.1683, 36.6301)
  point P59 (32.0697, 37.1)
  point P60 (29.9535, 38.4623)
  point P61 (29.8048, 38.5777)
  point P62 (29.6769, 39.0404)
  point P63 (30.2821, 41.0366)
  point P64 (27.9545, 40.2851)
  point P65 (27.4794, 40.2672)
  point P66 (27.3237, 40.373)
  point P67 (27.1669, 40.8268)
  point P68 (27.6457, 42.857)
  point P69 (24.8967, 41.9132)
  point P70 (24.7347, 42.009)
  point P71 (24.5498, 42.4521)
  point P72 (24.9001, 44.5083)
  point P73 (22.685, 43.471)
  point P74 (22.2159, 43.3938)
  point P75 (22.0481, 43.4792)
  point P76 (21.8358, 43.9098)
  point P77 (22.0563, 45.984)
  point P78 (19.4473, 44.7031)
  point P79 (19.2745, 44.7778)
  point P80 (19.0356, 45.1942)
  point P81 (19.1254, 47.2782)
  point P82 (16.602, 45.836)
  point P83 (16.4249, 45.8997)
  point P84 (16.1602, 46.3003)
  point P85 (13.6912, 46.788)